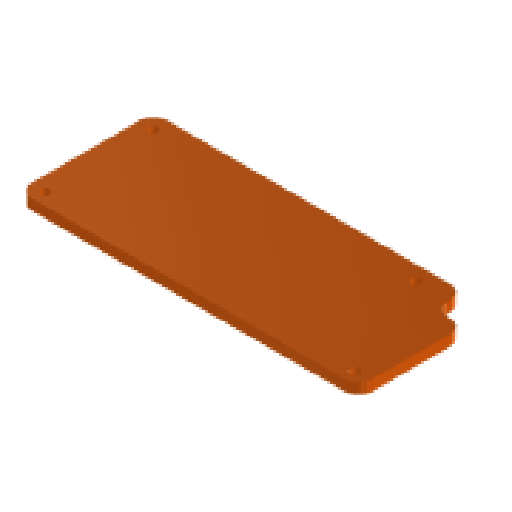
# Autodesk Inventor part: Frame_Foot_Solid
Saved by Autodesk Inventor 2023.2 (Build 272271000, 271)
## iProperties
Created: 2020-05-24
Part Number: Frame_Foot_Solid
Material: ABS Plastic
Document SubType Name: Modeling
Designer: Remo
Mass: 29.4079 g
Surface Area: 145.065 cm^2
Volume: 31.285 cm^3
Density: 1.06 g/cm^3
Appearance: Smooth - Light Orange
Description: 3DP Part / PET-G / Machine Foot - Mount Plate
Author: Remo
Revision Number: 1
Autodesk Inventor part; units mm, degrees
ref_plane "YZ Plane" through (0, 0, 0) normal (1, 0, 0) x (0, 1, 0)
ref_plane "XZ Plane" through (0, 0, 0) normal (0, 1, 0) x (-1, 0, 0)
ref_plane "XY Plane" through (0, 0, 0) normal (0, 0, 1) x (1, 0, 0)
sketch "Sketch1" plane through (0, 0, 0) normal (0, 0, 1) x (1, 0, 0)
  line L0 (0, 0) -> (0, 15)
  line L1 (0, 15) -> (-15, 15)
  line L2 (-15, 0) -> (-15, 15)
  line L3 (0, 0) -> (-15, 0)
  line L4 (-15, 15) -> (-515, 15)
  line L5 (-15, 0) -> (-515, 0)
  line L6 (-15, -360) -> (-15, 0)
  line L7 (0, -360) -> (0, 0)
  line L8 (-115, -360) -> (-115, 0)
  line L9 (-130, -360) -> (-130, 0)
  line L10 (-128, 13) -> (-2, 13)
  line L11 (-2, 13) -> (-2, -37)
  line L12 (-2, -37) -> (-128, -37)
  line L13 (-128, -37) -> (-128, 13)
  line L14 (-13, 13) -> (-13, 2)
  line L15 (-13, 2) -> (-2, 2)
extrude "Extrusion1" add sketch "Sketch1" along normal blind 4 contours L11 L12 L6 L3 | L3 L2 L10 L14 L15 L11 | L5 L13 L10 L2 | L6 L12 L8 L5 | L8 L12 L13 L5
sketch "Sketch2" plane through (0, 0, 4) normal (0, 0, 1) x (1, 0, 0)
  line L0 (-13, 13) -> (-128, 13) projected
  line L1 (-128, 13) -> (-128, -37) projected
  line L2 (-128, -37) -> (-2, -37) projected
  line L3 (-2, -37) -> (-2, 2) projected
  line L4 (-13, 2) -> (-13, 13) projected
  line L5 (-2, 2) -> (-13, 2) projected
  point P0 (0, 0)
  point P1 (-122.5, -32.4606)
  point P2 (-122.5, 7.5)
  point P3 (-25, 7.5)
  point P4 (-7.5, -32.4606)
  dimension "d6" = 5.5
  dimension "d7" = 5.5
  dimension "d8" = 5.5
  dimension "d9" = 23
  constraints: 1 horizontal alignment, 1 vertical alignment
  measures "d6" distance from line of L3 point (-7.5, -32.461)
  measures "d7" distance from line of L1 point (-122.5, -32.461)
  measures "d8" distance from line of L0 point (-122.5, 7.5)
  measures "d9" distance from line of L3 point (-25, 7.5)
hole "Hole1" at (-122.5, -32.4606, 4) at (-122.5, 7.5, 4) at (-25, 7.5, 4) at (-7.5, -32.4606, 4) direction (0, 0, -1) diameter 3.7 depth 8 tip angle 118
fillet "Fillet1" radius 5 6 edges at (-2, -37, 2) (-128, -37, 2) (-128, 13, 2) (-13, 13, 2) (-13, 2, 2) (-2, 2, 2)
equation "\"d7\" = d6"
equation "\"d8\" = d6"
equation "\"d1\" = d0"
equation "\"d3\" = d1"
equation "\"d21\" = d20"
equation "\"d0\" = 2"
equation "\"d20\" = 2"
body "Solid1"
